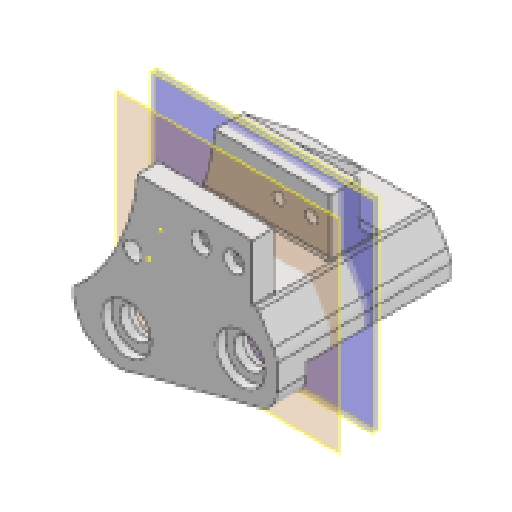
# Autodesk Inventor part: swingarmBaseV5
Saved by Autodesk Inventor 2025 (Build 290162000, 162)
## iProperties
Created: 2024-10-14
Part Number: swingarmBaseV5
Material: Generic
Document SubType Name: Modeling
Designer: derm
Density: 1 g/cm^3
Appearance: Default
Author: derm
Autodesk Inventor part; units mm, degrees
ref_plane "YZ Plane" through (0, 0, 0) normal (1, 0, 0) x (0, 1, 0)
ref_plane "XZ Plane" through (0, 0, 0) normal (0, 1, 0) x (-1, 0, 0)
ref_plane "XY Plane" through (0, 0, 0) normal (0, 0, 1) x (1, 0, 0)
sketch "Sketch1" plane through (0, 0, 0) normal (1, 0, 0) x (0, 1, 0)
  line L0 (-12.7635, 12.7635) -> (12.7635, 12.7635)
  line L1 (12.7635, 12.7635) -> (12.7635, -12.7635)
  line L2 (12.7635, -12.7635) -> (-12.7635, -12.7635)
  line L3 (-12.7635, -12.7635) -> (-12.7635, 12.7635)
  line L4 (-12.7635, 12.7635) -> (12.7635, -12.7635) construction
  line L5 (12.7635, 12.7635) -> (-12.7635, -12.7635) construction
  line L6 (19.1135, 19.1135) -> (-19.1135, 19.1135)
  line L7 (-19.1135, 19.1135) -> (-19.1135, -19.1135)
  line L8 (-19.1135, -19.1135) -> (19.1135, -19.1135)
  line L9 (19.1135, -19.1135) -> (19.1135, 19.1135)
  line L10 (12.7635, 19.1135) -> (12.7635, -19.1135)
  line L11 (-19.1135, -5.4793) -> (-46.5737, -5.4793)
  line L12 (-46.5737, -5.4793) -> (-46.5737, -19.1135)
  line L13 (-46.5737, -19.1135) -> (-19.1135, -19.1135)
  line L14 (-19.1135, -19.1135) -> (-19.1135, -5.4793)
  point P0 (0, 0)
  point P1 (12.7635, 12.7635)
  dimension "d1" = 25.527
  dimension "d2" = 6.35
  constraints: 30 end point, 6 parallel, 4 point on line, 3 perpendicular, 2 horizontal, 2 midpoint, 3 other
  measures "d1" distance of L1.end L2.end
  measures "d2" distance between parallel lines of L0 L6
extrude "Extrusion1" add sketch "Sketch1" along normal blind 50.8 contours L13 L12 L11 L7
sketch "Sketch2" plane through (0, -46.5737, -5.4793) normal (0, 0, 1) x (1, 0, 0)
  line L0 (0, 27.4602) -> (0, 0) projected
  line L1 (0, 0) -> (50.8, 0) projected
  line L2 (50.8, 27.4602) -> (50.8, 0) projected
  line L3 (0, 27.4602) -> (50.8, 27.4602) projected
  circle A0 centre (36.2123, 13.7301) radius 7
  point P0 (0, 46.5737)
  dimension "d5" = 14
  constraints: 1 centre point
  measures "d5" diameter of A0
extrude "Extrusion2" cut sketch "Sketch2" against normal through all contours A0
sketch "Sketch7" plane through (0, -46.5737, -5.4793) normal (0, 0, 1) x (1, 0, 0)
  circle A0 centre (36.2123, 13.7301) radius 7 projected
  circle A1 centre (36.2123, 13.7301) radius 11.1
  point P0 (0, 46.5737)
  dimension "d21" = 22.2
  constraints: 1 centre point, 1 coincident
  measures "d21" diameter of A1
extrude "Extrusion7" cut sketch "Sketch7" against normal blind 4
sketch "Sketch10" plane through (0, -46.5737, -19.1135) normal (0, 0, -1) x (-1, 0, 0)
  circle A0 centre (-36.2123, 13.7301) radius 7 projected
  line L0 (0, 0) -> (0, 27.4602) projected
  line L1 (0, 27.4602) -> (-50.8, 27.4602) projected
  line L2 (-50.8, 0) -> (-50.8, 27.4602) projected
  line L3 (0, 0) -> (-50.8, 0) projected
  circle A1 centre (-36.2123, 13.7301) radius 11
  point P0 (0, 46.5737)
  constraints: 1 centre point, 1 coincident
extrude "Extrusion10" cut sketch "Sketch10" against normal blind 5.5 contours A1
sketch "Sketch11" plane through (0, -46.5737, -5.4793) normal (0, 0, 1) x (1, 0, 0)
  circle A0 centre (36.2123, 13.7301) radius 11.1 projected
  circle A1 centre (8.2123, 21.7301) radius 2.6
  point P0 (0, 46.5737)
  dimension "d34" = 28
  dimension "d35" = 8
  dimension "d36" = 5.2
  constraints: 1 centre point
  measures "d34" horizontal distance of A0.centre A1.centre
  measures "d35" vertical distance of A0.centre A1.centre
  measures "d36" diameter of A1
extrude "Extrusion11" cut sketch "Sketch11" against normal through all contours A1
sketch "Sketch12" plane through (0, -19.1135, -5.4793) normal (0, 1, 0) x (1, 0, 0)
  line L0 (0, 13.6342) -> (0, 0) projected
  line L1 (0, 0) -> (50.8, 0) projected
  line L2 (50.8, 13.6342) -> (50.8, 0) projected
  line L3 (0, 13.6342) -> (50.8, 13.6342) projected
  point P0 (0, -5.4793)
extrude "Extrusion12" add sketch "Sketch12" along normal blind 10
sketch "Sketch13" plane through (50.8, -46.5737, -19.1135) normal (0, 0, -1) x (-1, 0, 0)
  circle A0 centre (42.5877, 21.7301) radius 2.6 projected
  circle A1 centre (14.5877, 13.7301) radius 11 projected
  line L0 (50.8, 0) -> (50.8, 37.4602) projected
  line L1 (0, 37.4602) -> (50.8, 37.4602) projected
  line L2 (0, 0) -> (0, 37.4602) projected
  line L3 (50.8, 0) -> (0, 0) projected
  line L4 (50.8, 0) -> (50.8, 37.4602) projected
  line L5 (0, 37.4602) -> (50.8, 37.4602)
  line L6 (50.8, 37.4602) -> (50.8, 28.3179)
  line L7 (50.8, 28.3179) -> (14.5877, 28.3179)
  line L8 (0, 28.3179) -> (0, 37.4602)
  arc A2 (14.5877, 28.3179) -> (0, 13.7301) centre (14.5877, 13.7301) ccw
  arc A3 (9.6596, 0) -> (19.5158, 0) centre (14.5877, 13.7301) ccw
  point P0 (50.8, 46.5737)
  constraints: 8 end point, 4 point on circle, 4 point on line, 2 centre point, 2 parallel, 2 tangent, 1 coincident, 1 horizontal, 1 perpendicular
extrude "Extrusion13" add sketch "Sketch13" along normal blind 26 contours L7 A2 L2 L1 L0
mirror "Mirror1" about plane through (25.4, -20.9786, -45.1135) normal (0, 0, -1)
fillet "Fillet5" [suppressed]
sketch "Sketch14" plane through (0, -9.1135, -5.4793) normal (0, 1, 0) x (1, 0, 0)
  line L0 (0, 0) -> (0, 79.2683) projected
  line L1 (0, 0) -> (50.8, 0) projected
  line L2 (50.8, 0) -> (50.8, 79.2683) projected
  line L3 (0, 79.2683) -> (50.8, 79.2683) projected
  circle A0 centre (-6.545, 39.6342) radius 15.197
  point P0 (0, -5.4793)
  constraints: 1 centre point
extrude "Extrusion14" cut sketch "Sketch14" against normal blind 26 contours A0 L0 | L0 A0
fillet "Fillet6" radius 10 2 edges at (0, -13.6847, -31.3981) (0, -13.6847, -58.8289)
sketch "Sketch15" plane through (50.8, -9.1135, -84.7477) normal (0, 0, -1) x (-1, 0, 0)
  line L0 (50.8, -37.4602) -> (0, -37.4602) projected
  line L1 (50.8, -37.4602) -> (50.8, 0) projected
  line L2 (50.8, 0) -> (0, 0) projected
  line L3 (0, -37.4602) -> (0, 0) projected
  circle A0 centre (42.5877, -15.7301) radius 2.6 projected
  circle A1 centre (14.5877, -23.7301) radius 11.1 projected
  circle A2 centre (-62.5324, 30.9366) radius 78.1359
  point P0 (50.8, 9.1135)
  point P1 (0, -15.9134)
  point P2 (9.2182, 0)
  constraints: 1 centre point
extrude "Extrusion15" cut sketch "Sketch15" against normal through all contours L3 L2 A2 picked at (1.1624, -8.9232)
thicken "Thicken1" operation add thickness 1.5 both sides no extend neighbours no toward (-0.9972038, -0.0747301, 0) faces at (50.7592, -31.7535, -36.4468)
fillet "Fillet7" radius 10 1 edges at (36.2123, -18.2559, -45.1135)
sketch "Sketch16" plane through (0, -9.1135, -5.4793) normal (0, 1, 0) x (1, 0, 0)
  line L0 (41.5818, 0) -> (41.5818, 79.2683) projected
  line L1 (0, 79.2683) -> (41.5818, 79.2683) projected
  line L2 (0, 58.6382) -> (0, 79.2683) projected
  arc A0 (0, 58.6382) -> (3.4337, 51.096) centre (10, 58.6382) ccw projected
  arc A1 (3.4337, 28.1723) -> (3.4337, 51.096) centre (-6.545, 39.6342) ccw projected
  arc A2 (3.4337, 28.1723) -> (0, 20.6301) centre (10, 20.6301) ccw projected
  line L3 (0, 0) -> (0, 20.6301) projected
  line L4 (0, 0) -> (41.5818, 0) projected
  line L5 (0, 0) -> (41.5818, 0)
  line L6 (41.5818, 0) -> (41.5818, 9.8)
  line L7 (41.5818, 9.8) -> (0, 9.8)
  line L8 (0, 9.8) -> (0, 0)
  line L9 (-402.451, 35.28) -> (156.349, 35.28) projected
  line L10 (8.0732, 35.48) -> (41.5818, 35.48)
  line L11 (5.8122, 48.48) -> (41.5818, 48.48)
  line L12 (41.5818, 48.48) -> (36.5818, 48.48)
  line L13 (36.5818, 48.48) -> (36.5818, 79.2683)
  line L14 (36.5818, 79.2683) -> (41.5818, 79.2683)
  line L15 (41.5818, 79.2683) -> (41.5818, 48.48)
  line L16 (5.8122, 48.48) -> (12.8122, 48.48)
  line L17 (12.8122, 48.48) -> (12.8122, 79.2683)
  line L18 (12.8122, 79.2683) -> (5.8122, 79.2683)
  line L19 (5.8122, 79.2683) -> (5.8122, 48.48)
  point P0 (0, -5.4793)
  point P1 (0, 9.8)
  dimension "d54" = 9.8
  dimension "d55" = 0.2
  dimension "d56" = 13
  dimension "d57" = 7
  dimension "d58" = 5
  constraints: 28 end point, 8 parallel, 5 point on line, 3 horizontal, 3 perpendicular, 2 point on circle
  measures "d54" distance between parallel lines of L4 L7
  measures "d55" distance between parallel lines of L9 L10
  measures "d56" distance between parallel lines of L10 L11
  measures "d57" distance between parallel lines of L19 L17
  measures "d58" distance between parallel lines of L0 L13
extrude "Extrusion16" add sketch "Sketch16" along normal blind 25.4 contours L4 L3 L7 L0 | L10 A1 L11 L0 | L19 L1 L17 L11
sketch "Sketch17" plane through (5.8122, -9.1135, -84.7477) normal (-1, 0, 0) x (0, 0, 1)
  line L0 (0, 0) -> (30.7883, 0) projected
  line L1 (0, 0) -> (0, 25.4) projected
  line L2 (30.7883, 25.4) -> (0, 25.4) projected
  line L3 (30.7883, 0) -> (30.7883, 25.4) projected
  line L4 (30.7883, 0) -> (0, 0) projected
  line L5 (30.7883, 0) -> (30.7883, 25.4) projected
  line L6 (0, 0) -> (30.7883, 25.4)
  point P0 (84.7477, 9.1135)
  constraints: 2 end point
extrude "Extrusion17" cut sketch "Sketch17" against normal blind 25.4 contours L1 L2 L6
fillet "Fillet8" radius 10 1 edges at (27.197, -9.1135, -53.9593)
sketch "Sketch18" plane through (-6.545, -18.2559, -45.1135) normal (0, -1, 0) x (1, 0, 0)
  line L0 (37.4895, 26) -> (37.4895, -26) projected
  line L1 (6.545, 26) -> (37.4895, 26) projected
  line L2 (6.545, 26) -> (6.545, 19.004) projected
  arc A0 (6.545, 19.004) -> (9.9788, 11.4619) centre (16.545, 19.004) ccw projected
  arc A1 (9.9788, -11.4619) -> (9.9788, 11.4619) centre (0, 0) ccw projected
  arc A2 (9.9788, -11.4619) -> (6.545, -19.004) centre (16.545, -19.004) ccw projected
  line L3 (6.545, -19.004) -> (6.545, -26) projected
  line L4 (6.545, -26) -> (37.4895, -26) projected
  line L5 (-395.906, 14.7702) -> (-395.906, 19.0981) projected
  line L6 (-395.906, 14.7702) -> (162.894, 14.7702) projected
  line L7 (162.894, 19.0981) -> (162.894, 14.7702) projected
  line L8 (-395.906, 19.0981) -> (162.894, 19.0981) projected
  circle A3 centre (29.9619, 16.9342) radius 2.6
  circle A4 centre (16.545, 16.9342) radius 2.6
  point P0 (6.545, 45.1135)
  dimension "d64" = 5.2
  constraints: 2 centre point
  measures "d64" diameter of A3
extrude "Extrusion18" cut sketch "Sketch18" against normal blind 25.4 contours A3 L6 L8 | L8 A3 | A3 L6 | A4 L8 | L8 A4 L6 | L6 A4
sketch "Sketch19" plane through (-6.545, -18.2559, -45.1135) normal (0, -1, 0) x (1, 0, 0)
  circle A0 centre (16.545, 16.9342) radius 2.6 projected
  circle A1 centre (29.9619, 16.9342) radius 2.6 projected
  circle A2 centre (16.545, 16.9342) radius 4
  circle A3 centre (29.9619, 16.9342) radius 4
  point P0 (6.545, 45.1135)
  dimension "d67" = 8
  dimension "d68" = 8
  constraints: 2 centre point, 2 coincident
  measures "d67" diameter of A3
  measures "d68" diameter of A2
extrude "Extrusion19" cut sketch "Sketch19" against normal blind 5
sketch "Sketch20" plane through (0, -46.5737, -84.7477) normal (0, 0, -1) x (-1, 0, 0)
  circle A0 centre (-8.2123, 21.7301) radius 2.6 projected
  circle A1 centre (-8.2123, 21.7301) radius 4.1
  point P0 (0, 46.5737)
  dimension "d71" = 8.2
  constraints: 1 centre point, 1 coincident
  measures "d71" diameter of A1
extrude "Extrusion20" cut sketch "Sketch20" against normal blind 8 contours A0 | A1
sketch "Sketch21" plane through (0, -46.5737, -5.4793) normal (0, 0, 1) x (1, 0, 0)
  circle A0 centre (8.2123, 21.7301) radius 2.6 projected
  circle A1 centre (8.2123, 21.7301) radius 4.1 projected
  circle A2 centre (8.2123, 21.7301) radius 3.5
  point P0 (0, 46.5737)
  dimension "d74" = 7
  constraints: 1 centre point, 1 coincident
  measures "d74" diameter of A2
extrude "Extrusion21" cut sketch "Sketch21" against normal blind 12 contours A2
sketch "Sketch22" plane through (41.5818, 16.2865, -53.9593) normal (0, 0, -1) x (-1, 0, 0)
  line L0 (444.0328, -10.536) -> (444.0328, -14.864) projected
  line L1 (444.0328, -10.536) -> (-114.7672, -10.536) projected
  line L2 (-114.7672, -14.864) -> (-114.7672, -10.536) projected
  line L3 (444.0328, -14.864) -> (-114.7672, -14.864) projected
  circle A0 centre (8.4648, -12.7) radius 2.6
  circle A1 centre (23.4097, -12.7) radius 2.6
  point P0 (41.5818, -16.2865)
  dimension "d77" = 5.2
  dimension "d78" = 5.2
  constraints: 2 centre point
  measures "d77" diameter of A0
  measures "d78" diameter of A1
extrude "Extrusion22" cut sketch "Sketch22" against normal through all contours A1 L3 L1 | L1 A1 | A1 L3 | A0 L3 L1 | L1 A0 | A0 L3
sketch "Sketch23" plane through (41.5818, 16.2865, -53.9593) normal (0, 0, -1) x (-1, 0, 0)
  circle A0 centre (23.4097, -12.7) radius 2.6 projected
  circle A1 centre (8.4648, -12.7) radius 2.6 projected
  line L0 (28.7696, -15.4) -> (0, -15.4) projected
  line L1 (28.7696, -15.4) -> (28.7696, 0) projected
  line L2 (0, 0) -> (28.7696, 0) projected
  line L3 (0, -15.4) -> (0, 0) projected
  circle A2 centre (8.4648, -12.7) radius 4.5
  circle A3 centre (23.4097, -12.7) radius 4.5
  point P0 (41.5818, -16.2865)
  dimension "d81" = 9
  dimension "d82" = 9
  constraints: 2 centre point, 2 coincident
  measures "d81" diameter of A3
  measures "d82" diameter of A2
extrude "Extrusion23" cut sketch "Sketch23" along normal mid plane 8 contours A0 | A3 L0 | L0 A3 | A2 L0 | L0 A2
ref_plane "Work Plane1" through (41.5818, -9.1135, -28.1193) normal (0, 0, -1) x (-1, 0, 0)
mirror "Mirror2" about plane through (41.5818, -9.1135, -28.1193) normal (0, 0, -1) of "Extrusion23"
fillet "Fillet9" [suppressed]
fillet "Fillet10" radius 5 1 edges at (50.8, -25.0269, -45.1135)
sketch "Sketch24" plane through (0, -46.5737, -84.7477) normal (0, -1, 0) x (1, 0, 0)
  line L0 (0, 79.2683) -> (0, 65.6342) projected
  line L1 (0, 65.6342) -> (50.8, 65.6342) projected
  line L2 (50.8, 79.2683) -> (50.8, 65.6342) projected
  line L3 (0, 79.2683) -> (50.8, 79.2683) projected
  line L4 (0, 0) -> (0, 13.6342) projected
  line L5 (0, 0) -> (50.8, 0) projected
  line L6 (50.8, 0) -> (50.8, 13.6342) projected
  line L7 (0, 13.6342) -> (50.8, 13.6342) projected
  point P0 (0, 84.7477)
extrude "Extrusion24" add sketch "Sketch24" along normal blind 5
sketch "Sketch25" plane through (41.5818, -9.1135, -84.7477) normal (0, 0, -1) x (-1, 0, 0)
  arc A0 (-8.2798, -14.634) -> (-9.2182, -17.5501) centre (-4.2182, -17.5501) ccw projected
  line L0 (-9.2182, -17.5501) -> (-9.2182, -42.4602) projected
  line L1 (41.5818, -42.4602) -> (-9.2182, -42.4602) projected
  line L2 (41.5818, -42.4602) -> (41.5818, 0) projected
  line L3 (41.5818, 0) -> (35.7696, 0) projected
  line L4 (35.7696, 0) -> (28.7696, 0) projected
  line L5 (28.7696, 0) -> (0, 0) projected
  arc A1 (-8.2798, -14.634) -> (0, 0) centre (-71.7506, 30.9366) ccw projected
  circle A2 centre (5.3695, -23.7301) radius 11.1 projected
  circle A3 centre (33.3695, -15.7301) radius 4.1 projected
  line L6 (5.3695, -42.4602) -> (41.5818, -27.5404)
  point P0 (41.5818, 9.1135)
  constraints: 2 end point, 2 point on line
extrude "Extrusion25" [suppressed]
fillet "Fillet12" [suppressed]
fillet "Fillet13" [suppressed]
chamfer "Chamfer2" distance 3 angle 45 5 edges at (0, -18.2559, -67.6155) (0.8988, -18.2559, -59.974) (8.652, -18.2559, -45.1135) (0.8988, -18.2559, -30.253) (0, -18.2559, -22.6115)
sketch "Sketch26" plane through (30.9444, -18.2559, -71.1135) normal (0, -1, 0) x (1, 0, 0)
  line L0 (-27.9444, 0) -> (-27.9444, 6.996) projected
  line L1 (-27.9444, 0) -> (0, 0) projected
  line L2 (0, 52) -> (0, 0) projected
  line L3 (-27.9444, 52) -> (0, 52) projected
  line L4 (-27.9444, 45.004) -> (-27.9444, 52) projected
  arc A0 (-27.9444, 45.004) -> (-25.5408, 39.7245) centre (-20.9444, 45.004) ccw projected
  arc A1 (-25.5408, 12.2755) -> (-25.5408, 39.7245) centre (-37.4895, 26) ccw projected
  arc A2 (-25.5408, 12.2755) -> (-27.9444, 6.996) centre (-20.9444, 6.996) ccw projected
  circle A3 centre (-7.5276, 42.9342) radius 4 projected
  circle A4 centre (-20.9444, 42.9342) radius 4 projected
  line L5 (-27.9444, 0) -> (-53.6411, 0)
  line L6 (-53.6411, 0) -> (-53.6411, 52)
  line L7 (-53.6411, 52) -> (-27.9444, 52)
  line L8 (-27.9444, 52) -> (-27.9444, 0)
  line L9 (10.6374, 55.8342) -> (-30.9444, 55.8342) projected
  line L10 (10.6374, 17.1542) -> (-18.1322, 17.1542) projected
  line L11 (-30.9444, 6.996) -> (-30.9444, -13.6342) projected
  line L12 (-30.9444, 55.8342) -> (-30.9444, 45.004) projected
  line L13 (-30.9444, 6.996) -> (-30.9444, 0) projected
  line L14 (-30.9444, 0) -> (-30.9444, 52)
  point P0 (-30.9444, 71.1135)
  point P1 (-30.9444, 54.8342)
  constraints: 10 end point, 2 parallel, 2 point on line, 1 horizontal, 1 perpendicular
extrude "Extrusion26" add sketch "Sketch26" against normal up to surface (9.1424 mm away) contours L5 L11 L14 L12 L7 L4 L8 L0 | L8 A0 A1 A2
sketch "Sketch27" plane through (0, -9.1135, -5.4793) normal (0, 1, 0) x (1, 0, 0)
  point P0 (0, -5.4793)
sketch "Sketch28" plane through (0, -9.1135, -5.4793) normal (0, 1, 0) x (1, 0, 0)
  line L0 (12.8122, 48.48) -> (5.8122, 48.48) projected
  arc A0 (8.0732, 35.48) -> (5.8122, 48.48) centre (-6.545, 39.6342) ccw projected
  line L1 (8.0732, 35.48) -> (41.5818, 35.48) projected
  line L2 (41.5818, 35.48) -> (41.5818, 48.48) projected
  line L3 (41.5818, 48.48) -> (12.8122, 48.48) projected
  line L4 (12.8122, 79.2683) -> (12.8122, 48.48) projected
  line L5 (5.8122, 79.2683) -> (12.8122, 79.2683) projected
  line L6 (5.8122, 48.48) -> (5.8122, 79.2683) projected
  line L7 (12.8122, 48.48) -> (5.8122, 48.48) projected
  line L8 (0, 9.8) -> (0, 79.2683) projected
  line L9 (0, 79.2683) -> (5.8122, 79.2683) projected
  line L10 (5.8122, 79.2683) -> (0, 79.2683)
  line L11 (8.0732, 35.48) -> (0, 35.48)
  point P0 (0, -5.4793)
  constraints: 4 end point, 1 horizontal, 1 perpendicular, 1 point on line
extrude "Extrusion27" add sketch "Sketch28" along normal up to surface (25.4 mm away) contours A0 L11 L8 L9 L6
sketch "Sketch29" plane through (5.8122, -9.1135, -84.7477) normal (1, 0, 0) x (0, 0, -1)
  line L0 (-30.7883, 25.4) -> (0, 0) projected
  line L1 (0, 0) -> (0, 25.4) projected
  line L2 (0, 25.4) -> (-30.7883, 25.4) projected
  point P0 (-84.7477, 9.1135)
extrude "Extrusion28" cut sketch "Sketch29" against normal blind 10
sketch "Sketch30" plane through (0, 0, 0) normal (-1, 0, 0) x (0, 0, 1)
  line L0 (-53.9593, 16.2865) -> (-84.7477, -9.1135) projected
  line L1 (-84.7477, -51.5737) -> (-84.7477, -9.1135) projected
  line L2 (-71.1135, -51.5737) -> (-84.7477, -51.5737) projected
  line L3 (-71.1135, -51.5737) -> (-71.1135, -18.2559) projected
  line L4 (-19.1135, -18.2559) -> (-71.1135, -18.2559) projected
  line L5 (-19.1135, -18.2559) -> (-19.1135, -51.5737) projected
  line L6 (-5.4793, -51.5737) -> (-19.1135, -51.5737) projected
  line L7 (-5.4793, -51.5737) -> (-5.4793, 16.2865) projected
  line L8 (-15.2793, 16.2865) -> (-5.4793, 16.2865) projected
  line L9 (-15.2793, -9.1135) -> (-15.2793, 16.2865) projected
  line L10 (-15.2793, -9.1135) -> (-40.9593, -9.1135) projected
  line L11 (-40.9593, -9.1135) -> (-40.9593, 16.2865) projected
  line L12 (-40.9593, 16.2865) -> (-53.9593, 16.2865) projected
  line L13 (-40.9593, -9.1135) -> (-63.9593, -9.1135) projected
  line L14 (-84.7477, -9.1135) -> (-63.9593, -9.1135) projected
  line L15 (-40.9593, -9.1135) -> (-84.7477, -9.1135)
  line L16 (-84.7477, -9.1135) -> (-5.4793, -9.1135)
  point P0 (0, 0)
  constraints: 4 end point, 2 point on line, 1 collinear
extrude "Extrusion29" add sketch "Sketch30" along normal blind 20 contours L14 L13 L10 L16 L7 L6 L5 L4 L3 L2 L1
pattern_linear "Rectangular Pattern1" [suppressed]
sketch "Sketch31" plane through (0.7123, -24.8436, -17.4793) normal (0, 0, 1) x (1, 0, 0)
  circle A0 centre (0, 0) radius 2.6 projected
  point P0 (-0.7123, 24.8436)
extrude "Extrusion30" [suppressed]
sketch "Sketch32" plane through (0, -9.1135, -5.4793) normal (0, 1, 0) x (1, 0, 0)
  line L0 (-20, 65.6342) -> (30.9444, 65.6342) projected
  line L1 (30.9444, 13.6342) -> (30.9444, 65.6342) projected
  line L2 (-20, 13.6342) -> (30.9444, 13.6342) projected
  line L3 (-20, 65.6342) -> (-20, 13.6342) projected
  circle A0 centre (23.4168, 22.7) radius 4 projected
  circle A1 centre (10, 22.7) radius 4 projected
  line L4 (-20, 65.6342) -> (-20, 13.6342) projected
  arc A2 (-20, 13.6342) -> (-20, 65.6342) centre (-29.611, 39.6342) ccw
  point P0 (0, -5.4793)
  constraints: 2 point on circle, 1 centre point
extrude "Extrusion31" cut sketch "Sketch32" against normal blind 10 contours A2 L3
sketch "Sketch33" plane through (0, -9.1135, -5.4793) normal (0, 1, 0) x (1, 0, 0)
  line L0 (0, 9.8) -> (0, 0) projected
  line L1 (0, 0) -> (41.5818, 0) projected
  line L2 (41.5818, 0) -> (41.5818, 9.8) projected
  line L3 (41.5818, 9.8) -> (0, 9.8) projected
  line L4 (12.8122, 48.48) -> (0, 48.48) projected
  line L5 (0, 9.8) -> (0, 0) projected
  line L6 (41.5818, 35.48) -> (0, 35.48) projected
  line L7 (41.5818, 35.48) -> (41.5818, 48.48) projected
  line L8 (41.5818, 48.48) -> (12.8122, 48.48) projected
  arc A0 (-20, 13.6342) -> (-20, 65.6342) centre (-29.611, 39.6342) ccw projected
  line L9 (-20, 0) -> (-20, 13.6342) projected
  line L10 (0, 0) -> (-20, 0) projected
  line L11 (0, 9.8) -> (0, 0) projected
  line L12 (0, 9.8) -> (41.5818, 9.8) projected
  line L13 (41.5818, 9.8) -> (41.5818, 35.48) projected
  line L14 (41.5818, 35.48) -> (0, 35.48) projected
  line L15 (0, 79.2683) -> (0, 35.48) projected
  line L16 (0, 79.2683) -> (-20, 79.2683) projected
  line L17 (-20, 65.6342) -> (-20, 79.2683) projected
  circle A1 centre (10, 22.7) radius 2.6 projected
  circle A2 centre (23.4168, 22.7) radius 2.6 projected
  line L18 (0, 9.8) -> (-20, 9.8)
  line L19 (0, 48.48) -> (-3.3408, 48.48)
  line L20 (0, 35.48) -> (-2.2046, 35.48)
  line L21 (0, 0) -> (41.5818, 0) projected
  line L22 (41.5818, 0) -> (41.5818, 9.8) projected
  line L23 (41.5818, 9.8) -> (0, 9.8) projected
  line L24 (0, 35.48) -> (0, 48.48) projected
  point P0 (0, -5.4793)
  constraints: 6 end point, 2 point on circle, 2 point on line, 1 parallel, 1 perpendicular
extrude "Extrusion32" add sketch "Sketch33" along normal up to surface (25.4 mm away) contours L3 L2 L1 L0 | L0 L10 L9 L18
fillet "Fillet14" radius 1 2 edges at (10.7909, -9.1135, -15.2793) (20.7909, -9.1135, -40.9593)
sketch "Sketch34" plane through (41.5818, -9.1135, -84.7477) normal (0, 0, -1) x (-1, 0, 0)
  line L0 (41.5818, 0) -> (28.7696, 0) projected
  line L1 (28.7696, 0) -> (0, 0) projected
  arc A0 (-8.2798, -14.634) -> (0, 0) centre (-71.7506, 30.9366) ccw projected
  arc A1 (-8.2798, -14.634) -> (-9.2182, -17.5501) centre (-4.2182, -17.5501) ccw projected
  line L2 (-9.2182, -17.5501) -> (-9.2182, -42.4602) projected
  line L3 (-9.2182, -42.4602) -> (61.5818, -42.4602) projected
  line L4 (61.5818, 0) -> (61.5818, -42.4602) projected
  line L5 (41.5818, 0) -> (61.5818, 0) projected
  circle A2 centre (33.3695, -15.7301) radius 4.1 projected
  line L6 (0, 10) -> (0, 0) projected
  line L7 (0, 0) -> (-2.106, 0)
  line L8 (-2.106, 0) -> (-11.1734, -14.634)
  line L9 (-11.1734, -14.634) -> (-11.1734, -42.4602)
  line L10 (-11.1734, -42.4602) -> (-9.2182, -42.4602)
  point P0 (41.5818, 9.1135)
  constraints: 8 end point, 2 perpendicular, 1 horizontal
extrude "Extrusion33" add sketch "Sketch34" against normal up to surface (79.2683 mm away) contours A0 A1 L2 L10 L9 L8 L7
sketch "Sketch35" plane through (50.8, -51.5737, -71.1135) normal (-1, 0, 0) x (0, 0, 1)
  line L0 (0, 0) -> (0, 18.7301) projected
  line L1 (0, 0) -> (52, 0) projected
  line L2 (52, 18.7301) -> (52, 0) projected
  line L3 (52, 18.7301) -> (0, 18.7301) projected
  point P0 (71.1135, 51.5737)
extrude "Extrusion34" cut sketch "Sketch35" against normal blind 10
fillet "Fillet15" [suppressed]
sketch "Sketch39" plane through (41.5818, -9.1135, -5.4793) normal (0, 0, 1) x (1, 0, 0)
  point P0 (-41.5818, 9.1135)
sketch "Sketch41" plane through (0, -46.5737, -76.7477) normal (0, 0, -1) x (-1, 0, 0)
  circle A0 centre (6.7877, 21.7301) radius 2.6 projected
  point P0 (0, 46.5737)
extrude "Extrusion39" cut sketch "Sketch41" against normal blind 10
sketch "Sketch42" plane through (-20, 0, 0) normal (-1, 0, 0) x (0, 0, 1)
  line L0 (-71.1135, -18.2559) -> (-71.1135, -9.1135) projected
  line L1 (-71.1135, -9.1135) -> (-84.7477, -9.1135) projected
  line L2 (-84.7477, -9.1135) -> (-84.7477, -51.5737) projected
  line L3 (-84.7477, -51.5737) -> (-71.1135, -51.5737) projected
  line L4 (-71.1135, -51.5737) -> (-71.1135, -18.2559) projected
  line L5 (-13.6135, -43.8436) -> (-13.6135, -21.8436) projected
  line L6 (-19.1135, -9.1135) -> (-19.1135, -18.2559) projected
  line L7 (-19.1135, -18.2559) -> (-19.1135, -51.5737) projected
  line L8 (-19.1135, -51.5737) -> (-5.4793, -51.5737) projected
  line L9 (-5.4793, -51.5737) -> (-5.4793, 16.2865) projected
  line L10 (-5.4793, 16.2865) -> (-15.2793, 16.2865) projected
  line L11 (-15.2793, -8.1135) -> (-15.2793, 16.2865) projected
  arc A0 (-16.2793, -9.1135) -> (-15.2793, -8.1135) centre (-16.2793, -8.1135) ccw projected
  line L12 (-16.2793, -9.1135) -> (-19.1135, -9.1135) projected
  line L13 (-84.7477, -23.7475) -> (-84.7477, -51.5737) projected
  line L14 (-84.7477, -51.5737) -> (-71.1135, -51.5737)
  line L15 (-71.1135, -51.5737) -> (-71.1135, -67.9032)
  line L16 (-71.1135, -67.9032) -> (-84.7477, -67.9032)
  line L17 (-84.7477, -67.9032) -> (-84.7477, -51.5737)
  line L18 (-19.1135, -51.5737) -> (-5.4793, -51.5737)
  line L19 (-5.4793, -51.5737) -> (-5.4793, -67.9032)
  line L20 (-5.4793, -67.9032) -> (-19.1135, -67.9032)
  line L21 (-19.1135, -67.9032) -> (-19.1135, -51.5737)
  point P0 (0, 0)
  constraints: 16 end point, 4 parallel, 2 horizontal, 2 perpendicular, 1 point on line
extrude "Extrusion40" add sketch "Sketch42" against normal up to surface (72.7552 mm away) contours L15 L16 L17 L3 | L8 L19 L20 L21
sketch "Sketch46" plane through (-20, 0, 0) normal (-1, 0, 0) x (0, 0, 1)
  line L0 (-71.1135, -18.2559) -> (-71.1135, -9.1135) projected
  line L1 (-71.1135, -9.1135) -> (-84.7477, -9.1135) projected
  line L2 (-84.7477, -9.1135) -> (-84.7477, -67.9032) projected
  line L3 (-84.7477, -67.9032) -> (-71.1135, -67.9032) projected
  line L4 (-71.1135, -67.9032) -> (-71.1135, -18.2559) projected
  line L5 (-19.1135, -9.1135) -> (-19.1135, -18.2559) projected
  line L6 (-19.1135, -18.2559) -> (-19.1135, -67.9032) projected
  line L7 (-19.1135, -67.9032) -> (-5.4793, -67.9032) projected
  line L8 (-5.4793, -67.9032) -> (-5.4793, 16.2865) projected
  line L9 (-5.4793, 16.2865) -> (-15.2793, 16.2865) projected
  line L10 (-15.2793, -8.1135) -> (-15.2793, 16.2865) projected
  arc A0 (-16.2793, -9.1135) -> (-15.2793, -8.1135) centre (-16.2793, -8.1135) ccw projected
  line L11 (-16.2793, -9.1135) -> (-19.1135, -9.1135) projected
  point P0 (0, 0)
extrude "Extrusion44" add sketch "Sketch46" along normal blind 20
sketch "Sketch43" plane through (12.8122, -9.1135, -84.7477) normal (0, 0, -1) x (-1, 0, 0)
  line L0 (12.8122, 0) -> (0, 0) projected
  line L1 (0, 0) -> (-30.8757, 0) projected
  line L2 (-30.8757, 0) -> (-39.943, -14.634) projected
  line L3 (-39.943, -14.634) -> (-39.943, -58.7897) projected
  line L4 (52.8122, -58.7897) -> (-39.943, -58.7897) projected
  line L5 (12.8122, 0) -> (52.8122, 0) projected
  circle A0 centre (4.5999, -15.7301) radius 4.1 projected
  circle A1 centre (28.5229, -37.9631) radius 11.1
  line L6 (52.8122, 0) -> (52.8122, -58.7897) projected
  point P0 (12.8122, 9.1135)
  dimension "d143" = 22.2
  constraints: 1 centre point
  measures "d143" diameter of A1
extrude "Extrusion41" cut sketch "Sketch43" against normal up to surface (4 mm away) contours A1
sketch "Sketch44" plane through (-15.7107, -47.0766, -80.7477) normal (0, 0, -1) x (-1, 0, 0)
  circle A0 centre (0, 0) radius 11.1 projected
  circle A1 centre (0, 0) radius 7
  point P0 (-15.7107, 47.0766)
  dimension "d148" = 14
  constraints: 1 centre point, 1 coincident
  measures "d148" diameter of A1
extrude "Extrusion42" cut sketch "Sketch44" against normal up to surface (9.6342 mm away) contours A1
sketch "Sketch45" plane through (-20, -18.2559, -71.1135) normal (0, 0, 1) x (1, 0, 0)
  circle A0 centre (4.2893, -28.8208) radius 7 projected
  circle A1 centre (4.2893, -28.8208) radius 11.1 projected
  point P0 (20, 18.2559)
extrude "Extrusion43" cut sketch "Sketch45" against normal up to surface (5.5 mm away)
ref_plane "Work Plane2" through (12.8122, -9.1135, -45.1135) normal (0, 0, -1) x (-1, 0, 0)
mirror "Mirror3" about plane through (12.8122, -9.1135, -45.1135) normal (0, 0, -1) of "Extrusion43", "Extrusion42", "Extrusion41", "Extrusion20", "Extrusion21", "Extrusion11"
sketch "Sketch47" plane through (41.5818, -9.1135, -5.4793) normal (0, 0, 1) x (1, 0, 0)
  line L0 (11.1734, -58.7897) -> (-81.5818, -58.7897) projected
  line L1 (11.1734, -14.634) -> (11.1734, -58.7897) projected
  line L2 (2.106, 0) -> (11.1734, -14.634) projected
  line L3 (0, 0) -> (2.106, 0) projected
  line L4 (0, 0) -> (0, 25.4) projected
  line L5 (0, 25.4) -> (-81.5818, 25.4) projected
  line L6 (-81.5818, -58.7897) -> (-81.5818, 25.4) projected
  circle A0 centre (-5.3695, -23.7301) radius 11.1 projected
  circle A1 centre (-57.2925, -37.9631) radius 11.1 projected
  circle A2 centre (-33.3695, -15.7301) radius 4.1 projected
  line L7 (-81.5818, -58.7897) -> (11.1734, -58.7897)
  line L8 (11.1734, -14.634) -> (11.1734, -58.7897)
  line L9 (-81.5818, -58.7897) -> (11.1734, -58.7897) projected
  line L10 (-73.3351, -58.7897) -> (11.1734, -36.7118)
  point P0 (-41.5818, 9.1135)
  point P1 (11.1734, -36.7118)
  point P2 (-73.3351, -58.7897)
  constraints: 6 end point, 2 collinear, 1 midpoint, 1 point on line
extrude "Extrusion45" cut sketch "Sketch47" against normal through all contours L0 L10 L1
sketch "Sketch49" plane through (12.8122, -9.1135, -84.7477) normal (0, 0, -1) x (-1, 0, 0)
  circle A0 centre (4.5999, -15.7301) radius 4.1 projected
  circle A1 centre (-23.4001, -23.7301) radius 11.1 projected
  line L0 (-39.943, -36.7118) -> (44.5655, -58.7897) projected
  line L1 (52.8122, -58.7897) -> (44.5655, -58.7897) projected
  line L2 (52.8122, 0) -> (52.8122, -58.7897) projected
  line L3 (12.8122, 0) -> (52.8122, 0) projected
  line L4 (12.8122, 0) -> (0, 0) projected
  line L5 (0, 0) -> (-30.8757, 0) projected
  line L6 (-30.8757, 0) -> (-39.943, -14.634) projected
  line L7 (-39.943, -14.634) -> (-39.943, -36.7118) projected
  circle A2 centre (28.5229, -37.9631) radius 11.1 projected
  circle A3 centre (25.5999, -5.7301) radius 2.6
  circle A4 centre (4.5999, -15.7301) radius 3.5 projected
  circle A5 centre (4.5999, -15.7301) radius 2.6 projected
  point P0 (12.8122, 9.1135)
  dimension "d162" = 21
  dimension "d164" = 10
  constraints: 1 centre point, 1 equal radius
  measures "d162" horizontal distance of A3.centre A0.centre
  measures "d164" vertical distance of A3.centre A0.centre
extrude "Extrusion46" cut sketch "Sketch49" against normal through all contours A3
sketch "Sketch50" plane through (12.8122, -9.1135, -84.7477) normal (0, 0, -1) x (-1, 0, 0)
  circle A0 centre (4.5999, -15.7301) radius 4.1 projected
  circle A1 centre (25.5999, -5.7301) radius 2.6 projected
  circle A2 centre (25.5999, -5.7301) radius 4.1
  point P0 (12.8122, 9.1135)
  dimension "d165" = 8.2
  constraints: 1 centre point, 1 coincident
  measures "d165" diameter of A2
extrude "Extrusion47" cut sketch "Sketch50" against normal blind 7 contours A2
ref_plane "Work Plane3" through (12.8122, -9.1135, -45.1135) normal (0, 0, -1) x (-1, 0, 0)
mirror "Mirror4" about plane through (12.8122, -9.1135, -45.1135) normal (0, 0, -1) of "Extrusion47"
ref_plane "Work Plane4" through (41.5818, -9.1135, -29.7193) normal (0, 0, 1) x (1, 0, 0)
mirror "Mirror5" about plane through (41.5818, -9.1135, -29.7193) normal (0, 0, 1) of "Extrusion23", "Extrusion22"
sketch "Sketch51" plane through (30.9444, -18.2559, -71.1135) normal (0, -1, 0) x (1, 0, 0)
  circle A0 centre (-20.9444, 42.9342) radius 4 projected
  circle A1 centre (-7.5276, 42.9342) radius 4 projected
  arc A2 (-50.9444, 0) -> (-50.9444, 52) centre (-60.5555, 26) ccw projected
  line L0 (-50.9444, 0) -> (0, 0) projected
  line L1 (0, 52) -> (0, 0) projected
  line L2 (-50.9444, 52) -> (0, 52) projected
  line L3 (-20.5332, 35.9231) -> (-45.3247, 35.9231)
  line L4 (-45.3247, 35.9231) -> (-45.3247, 11.5388)
  line L5 (-45.3247, 11.5388) -> (-20.5332, 11.5388)
  line L6 (-20.5332, 11.5388) -> (-20.5332, 35.9231)
  line L7 (-20.5332, 35.9231) -> (-45.3247, 11.5388) construction
  line L8 (-45.3247, 35.9231) -> (-20.5332, 11.5388) construction
  line L9 (-32.929, 11.5388) -> (-32.929, 35.9231)
  point P0 (-30.9444, 71.1135)
  point P1 (-32.929, 23.7309)
  point P2 (-34.6729, 35.9231)
  point P3 (-36.9071, 11.5388)
  constraints: 14 end point, 4 midpoint, 2 parallel, 1 horizontal, 1 perpendicular, 1 point on circle, 1 other
sketch "Sketch52" plane through (30.9444, -18.2559, -19.1135) normal (0, 0, -1) x (-1, 0, 0)
  circle A0 centre (22.7322, -6.5877) radius 2.6 projected
  circle A1 centre (-5.2678, -14.5877) radius 11 projected
  line L0 (-21.8108, -27.5694) -> (62.6977, -49.6473) projected
  line L1 (62.6977, -49.6473) -> (70.9444, -49.6473) projected
  line L2 (70.9444, 9.1424) -> (70.9444, -49.6473) projected
  line L3 (50.9444, 9.1424) -> (70.9444, 9.1424) projected
  line L4 (50.9444, 9.1424) -> (50.9444, 0) projected
  line L5 (50.9444, 0) -> (0, 0) projected
  arc A2 (0, 0) -> (-5.2678, -1.5) centre (0, -10) ccw projected
  arc A3 (-5.2678, -1.5) -> (-18.3556, -14.5877) centre (-5.2678, -14.5877) ccw projected
  line L6 (-18.3556, -14.5877) -> (-21.8108, -14.5877) projected
  line L7 (-21.8108, -27.5694) -> (-21.8108, -14.5877) projected
  circle A4 centre (46.6552, -28.8208) radius 11.1 projected
  spline S0 degree 2 poles (46.3322, 3.4123) (46.3322, 7.9156) (42.4322, 5.6639) (38.5322, 3.4123) (42.4322, 1.1606) (46.3322, -1.0911) (46.3322, 3.4123) knots 0 0 0 0.333333 0.333333 0.666667 0.666667 1 1 1 weights 1 0.5 1 0.5 1 0.5 1 projected
  line L8 (50.9444, 0) -> (50.9444, 0) projected
  line L9 (50.9444, 9.1424) -> (50.9444, 0) projected
  line L10 (50.9444, 9.1424) -> (50.9444, 9.1424) projected
  line L11 (50.9444, 0) -> (50.9444, 9.1424) projected
  line L12 (36.9815, 0) -> (36.9815, 9.1424)
  line L13 (36.9815, 9.1424) -> (50.9444, 9.1424)
  line L14 (-10.6374, 9.1424) -> (70.9444, 9.1424) projected
  line L15 (34.7197, 4) -> (34.7197, 9.1424)
  line L16 (50.9444, 9.1424) -> (60.5203, 9.1424)
  line L17 (60.5203, 9.1424) -> (60.5203, 0)
  line L18 (60.5203, 0) -> (50.9444, 0)
  line L19 (50.9444, 0) -> (50.9444, 9.1424)
  line L20 (27.5865, 9.1424) -> (27.5865, 0)
  point P0 (30.9444, 18.2559)
  point P1 (60.5203, 9.1424)
  constraints: 16 end point, 3 point on line, 2 parallel, 2 perpendicular, 1 collinear, 1 horizontal, 1 vertical, 3 other
extrude "Extrusion49" add sketch "Sketch52" along normal blind 21 contours L17 L18 L4 L3 | L4 L5 L12 L13 | L20 L14 L12 L5
ref_plane "Work Plane5" through (14.8297, -14.2559, -47.3826) normal (0, 0, -1) x (-1, 0, 0)
mirror "Mirror6" about plane through (14.8297, -14.2559, -47.3826) normal (0, 0, -1) of "Extrusion49"
sketch "Sketch53" plane through (30.9444, -18.2559, -71.1135) normal (0, -1, 0) x (1, 0, 0)
  line L0 (-60.5203, 0) -> (0, 0) projected
  line L1 (0, 52) -> (0, 0) projected
  line L2 (-60.5203, 52) -> (0, 52) projected
  line L3 (-60.5203, 52) -> (-60.5203, 31) projected
  line L4 (-33.2906, 31) -> (-60.5203, 31) projected
  line L5 (-34.5286, 16.4619) -> (-60.5203, 16.4619) projected
  line L6 (-60.5203, 0) -> (-60.5203, 16.4619) projected
  circle A0 centre (-7.5276, 42.9342) radius 4 projected
  circle A1 centre (-20.9444, 42.9342) radius 4 projected
  line L7 (0, 52) -> (5.2678, 52) projected
  line L8 (0, 52) -> (0, 0) projected
  line L9 (5.2678, 0) -> (0, 0) projected
  line L10 (5.2678, 52) -> (5.2678, 0) projected
  line L11 (5.2678, 52) -> (18.3556, 52) projected
  line L12 (5.2678, 52) -> (5.2678, 0) projected
  line L13 (18.3556, 0) -> (5.2678, 0) projected
  line L14 (18.3556, 52) -> (18.3556, 0) projected
  arc A2 (-34.5286, 16.4619) -> (-33.2906, 31) centre (-60.5555, 26) ccw projected
  point P0 (-30.9444, 71.1135)
extrude "Extrusion50" [suppressed]
sketch "Sketch54" plane through (12.8122, -9.1135, -84.7477) normal (0, 0, -1) x (-1, 0, 0)
  circle A0 centre (25.5999, -5.7301) radius 4.1 projected
  circle A1 centre (4.5999, -15.7301) radius 4.1 projected
  circle A2 centre (-23.4001, -23.7301) radius 11.1 projected
  line L0 (-39.943, -36.7118) -> (44.5655, -58.7897) projected
  line L1 (52.8122, -58.7897) -> (44.5655, -58.7897) projected
  line L2 (52.8122, 0) -> (52.8122, -58.7897) projected
  line L3 (12.8122, 0) -> (52.8122, 0) projected
  line L4 (12.8122, 0) -> (0, 0) projected
  line L5 (0, 0) -> (-30.8757, 0) projected
  line L6 (-30.8757, 0) -> (-39.943, -14.634) projected
  line L7 (-39.943, -14.634) -> (-39.943, -36.7118) projected
  circle A3 centre (28.5229, -37.9631) radius 11.1 projected
  line L8 (52.8122, -16.7272) -> (-19.9536, -41.9341)
  point P0 (12.8122, 9.1135)
  constraints: 2 end point, 2 point on line
extrude "Extrusion51" cut sketch "Sketch54" against normal blind 15 contours L8 L2 L1 L0 | A3
fillet "Fillet21" radius 2 1 edges at (43.6878, -9.1135, -45.1135)
fillet "Fillet22" radius 10 1 edges at (52.7552, -23.7475, -45.1135)
fillet "Fillet23" radius 10 2 edges at (52.7552, -45.8253, -12.2964) (52.7552, -45.8253, -77.9306)
fillet "Fillet24" radius 40 1 edges at (32.7657, -51.0476, -77.9306)
fillet "Fillet26" radius 20 2 edges at (-31.7533, -67.9032, -12.2964) (-40, -67.9032, -12.2964)
sketch "Sketch55" plane through (52.7552, -32.8436, -19.1135) normal (0, 0, -1) x (-1, 0, 0)
  circle A0 centre (16.5429, 0) radius 11.1 projected
  circle A1 centre (44.5429, 8) radius 4.1 projected
  circle A2 centre (65.5429, 18) radius 4.1 projected
  arc A3 (8.2503, -15.1371) -> (31.4541, -14.2324) centre (18.361, 23.564) ccw projected
  line L0 (31.4541, -14.2324) -> (92.7552, 7.003) projected
  line L1 (92.7552, 23.7301) -> (92.7552, 7.003) projected
  line L2 (52.7552, 23.7301) -> (92.7552, 23.7301) projected
  line L3 (52.7552, 23.7301) -> (39.943, 23.7301) projected
  line L4 (39.943, 23.7301) -> (10.1809, 23.7301) projected
  arc A4 (10.1809, 23.7301) -> (8.4808, 22.7835) centre (10.1809, 21.7301) ccw projected
  line L5 (8.4808, 22.7835) -> (1.4995, 11.5162) projected
  arc A5 (1.4995, 11.5162) -> (0, 6.2492) centre (10, 6.2492) ccw projected
  line L6 (0, 6.2492) -> (0, -5.2586) projected
  arc A6 (0, -5.2586) -> (7.4723, -14.9338) centre (10, -5.2586) ccw projected
  line L7 (7.4723, -14.9338) -> (8.2503, -15.1371) projected
  line L8 (82.331, 23.7301) -> (82.331, 14.5877) projected
  line L9 (82.331, 23.7301) -> (92.7552, 23.7301)
  line L10 (92.7552, 23.7301) -> (92.7552, 7.003)
  line L11 (92.7552, 7.003) -> (82.331, 7.003)
  line L12 (82.331, 7.003) -> (82.331, 23.7301)
  point P0 (52.7552, 32.8436)
  point P1 (82.331, 12.5877)
  constraints: 8 end point, 2 parallel, 1 horizontal, 1 perpendicular
extrude "Extrusion52" add sketch "Sketch55" along normal up to surface (52 mm away) contours L11 L12 L8 L2 L1
sketch "Sketch56" plane through (12.8122, -9.1135, -84.7477) normal (0, 0, -1) x (-1, 0, 0)
  circle A0 centre (-23.4001, -23.7301) radius 11.1 projected
  circle A1 centre (4.5999, -15.7301) radius 4.1 projected
  circle A2 centre (25.5999, -5.7301) radius 4.1 projected
  arc A3 (-31.6927, -38.8672) -> (-8.4889, -37.9626) centre (-21.582, -0.1661) ccw projected
  line L0 (-8.4889, -37.9626) -> (52.8122, -16.7272) projected
  line L1 (52.8122, 0) -> (52.8122, -16.7272) projected
  line L2 (12.8122, 0) -> (52.8122, 0) projected
  line L3 (12.8122, 0) -> (0, 0) projected
  line L4 (0, 0) -> (-29.7621, 0) projected
  arc A4 (-29.7621, 0) -> (-31.4622, -0.9466) centre (-29.7621, -2) ccw projected
  line L5 (-31.4622, -0.9466) -> (-38.4435, -12.2139) projected
  arc A5 (-38.4435, -12.2139) -> (-39.943, -17.4809) centre (-29.943, -17.4809) ccw projected
  line L6 (-39.943, -17.4809) -> (-39.943, -28.9887) projected
  arc A6 (-39.943, -28.9887) -> (-32.4707, -38.664) centre (-29.943, -28.9887) ccw projected
  line L7 (-32.4707, -38.664) -> (-31.6927, -38.8672) projected
  line L8 (-39.943, -23.7301) -> (32.5965, -23.7301)
  point P0 (12.8122, 9.1135)
  constraints: 2 end point, 1 horizontal, 1 point on line
extrude "Extrusion53" cut sketch "Sketch56" against normal up to surface (13.6342 mm away) contours L8 L0 A3 L7 A6 L6 A0 | A0 L8 picked at (-24.7121, -27.1897)
sketch "Sketch57" plane through (12.8122, -9.1135, -84.7477) normal (0, 0, -1) x (-1, 0, 0)
  arc A0 (-12.3001, -23.7301) -> (-34.5001, -23.7301) centre (-23.4001, -23.7301) ccw projected
  circle A1 centre (-23.4001, -23.7301) radius 11.8982
  line L0 (-35.2982, -23.7301) -> (-11.5019, -23.7301)
  line L1 (32.5965, -23.7301) -> (-12.4001, -23.7301) projected
  point P0 (12.8122, 9.1135)
  point P1 (-28.7696, 25.4)
  constraints: 2 end point, 2 point on circle, 1 centre point, 1 coincident, 1 point on line
extrude "Extrusion54" add sketch "Sketch57" against normal up to surface (8.1342 mm away) contours L0 A0 | A0 L0 A1
sketch "Sketch58" plane through (12.8122, -9.1135, -84.7477) normal (0, 0, -1) x (-1, 0, 0)
  circle A0 centre (4.5999, -15.7301) radius 4.1 projected
  circle A1 centre (25.5999, -5.7301) radius 4.1 projected
  line L0 (-39.943, -23.7301) -> (32.5965, -23.7301) projected
  line L1 (32.5965, -23.7301) -> (52.8122, -16.7272) projected
  line L2 (52.8122, 0) -> (52.8122, -16.7272) projected
  line L3 (12.8122, 0) -> (52.8122, 0) projected
  line L4 (12.8122, 0) -> (0, 0) projected
  line L5 (0, 0) -> (-29.7621, 0) projected
  arc A2 (-29.7621, 0) -> (-31.4622, -0.9466) centre (-29.7621, -2) ccw projected
  line L6 (-31.4622, -0.9466) -> (-38.4435, -12.2139) projected
  arc A3 (-38.4435, -12.2139) -> (-39.943, -17.4809) centre (-29.943, -17.4809) ccw projected
  line L7 (-39.943, -17.4809) -> (-39.943, -23.7301) projected
  circle A4 centre (110.762, 31.5977) radius 87.2843
  point P0 (12.8122, 9.1135)
  dimension "d189" = 57.9498
  dimension "d190" = 31.5977
  constraints: 1 centre point
  measures "d189" distance from line of A4.centre L2
  measures "d190" distance from line of A4.centre L3
extrude "Extrusion55" cut sketch "Sketch58" against normal through all contours A4 L3 L2 L1 | L1 L2 L3 A4
extrude "Extrusion57" cut sketch "Sketch51" against normal blind 4 contours A2 L9 L5 | A2 L9 L3 L6 L5 | A2 L3 L9
sketch "Sketch59" plane through (12.8122, -9.1135, -84.7477) normal (0, 0, -1) x (-1, 0, 0)
  arc A0 (29.3978, 0) -> (40.9756, -20.8275) centre (110.762, 31.5977) ccw projected
  line L0 (12.8122, 0) -> (29.3978, 0) projected
  line L1 (12.8122, 0) -> (0, 0) projected
  line L2 (0, 0) -> (-29.7621, 0) projected
  arc A1 (-29.7621, 0) -> (-31.4622, -0.9466) centre (-29.7621, -2) ccw projected
  line L3 (-31.4622, -0.9466) -> (-38.4435, -12.2139) projected
  arc A2 (-38.4435, -12.2139) -> (-39.943, -17.4809) centre (-29.943, -17.4809) ccw projected
  line L4 (-39.943, -17.4809) -> (-39.943, -23.7301) projected
  line L5 (-39.943, -23.7301) -> (32.5965, -23.7301) projected
  line L6 (32.5965, -23.7301) -> (40.9756, -20.8275) projected
  circle A3 centre (4.5999, -15.7301) radius 4.1 projected
  circle A4 centre (25.5999, -5.7301) radius 4.1 projected
  point P0 (12.8122, 9.1135)
extrude "Extrusion58" add sketch "Sketch59" against normal up to surface (13.6342 mm away) contours A3
sketch "Sketch60" plane through (41.5818, -9.1135, -5.4793) normal (0, 0, 1) x (1, 0, 0)
  circle A0 centre (-33.3695, -15.7301) radius 4.1 projected
  point P0 (-41.5818, 9.1135)
extrude "Extrusion59" add sketch "Sketch60" against normal up to surface (13.6342 mm away)
sketch "Sketch61" plane through (0, 0, 0) normal (-1, 0, 0) x (0, 0, 1)
  line L0 (-84.7477, -9.1135) -> (-39.9593, -9.1135) projected
  arc A0 (-40.9593, -8.1135) -> (-39.9593, -9.1135) centre (-39.9593, -8.1135) ccw projected
  line L1 (-40.9593, -8.1135) -> (-40.9593, 16.2865) projected
  line L2 (-40.9593, 16.2865) -> (-53.9593, 16.2865) projected
  line L3 (-53.9593, 16.2865) -> (-84.7477, -9.1135) projected
  point P0 (0, 0)
extrude "Extrusion60" add sketch "Sketch61" along normal up to surface round surface about axis through (-97.9498, 22.4842, -84.7477) along (0, 0, 1) radius 87.2843 far side no
sketch "Sketch62" plane through (52.7552, -32.8436, -84.7477) normal (0, 0, -1) x (-1, 0, 0)
  arc A0 (63.641, 49.1301) -> (69.3408, 23.7301) centre (150.705, 55.3278) ccw projected
  arc A1 (69.3408, 23.7301) -> (80.9186, 2.9026) centre (150.705, 55.3278) ccw projected
  arc A2 (73.5118, 14.5877) -> (92.7552, -9.9437) centre (150.705, 55.3278) ccw projected
  arc A3 (63.641, 49.1301) -> (92.7552, -9.9437) centre (150.705, 55.3278) ccw
  line L0 (57.0451, 49.1301) -> (90.2775, -20.9598)
  line L1 (39.943, 23.7301) -> (39.943, 49.1301) projected
  line L2 (39.943, 23.7301) -> (69.3408, 23.7301) projected
  arc A4 (63.641, 49.1301) -> (69.3408, 23.7301) centre (150.705, 55.3278) ccw projected
  line L3 (39.943, 49.1301) -> (63.641, 49.1301) projected
  arc A5 (73.5118, 14.5877) -> (92.7552, -9.9437) centre (150.705, 55.3278) ccw projected
  line L4 (73.5118, 14.5877) -> (21.8108, 14.5877) projected
  arc A6 (21.8108, 14.5877) -> (16.5429, 13.0877) centre (21.8108, 4.5877) ccw projected
  arc A7 (16.5429, 13.0877) -> (3.4552, 0) centre (16.5429, 0) ccw projected
  line L5 (3.4552, 0) -> (0, 0) projected
  line L6 (0, -5.2586) -> (0, 0) projected
  arc A8 (0, -5.2586) -> (7.4723, -14.9338) centre (10, -5.2586) ccw projected
  line L7 (7.4723, -14.9338) -> (67.6998, -30.6683) projected
  arc A9 (67.6998, -30.6683) -> (92.7552, -11.3177) centre (72.7552, -11.3177) ccw projected
  line L8 (92.7552, -9.9437) -> (92.7552, -11.3177) projected
  circle A10 centre (16.5429, 0) radius 11 projected
  circle A11 centre (68.4659, -14.233) radius 11.1 projected
  point P0 (52.7552, 32.8436)
  point P1 (92.7552, -9.9437)
  point P2 (73.5118, 14.5877)
  point P3 (73.423, 14.5877)
  point P4 (63.641, 49.1301)
  point P5 (69.0883, 23.7301)
  point P6 (69.3408, 23.7301)
  point P7 (71.8367, 17.9333)
  point P8 (69.3408, 23.7301)
  constraints: 4 end point, 4 point on circle, 1 centre point, 1 coincident, 1 point on line, 1 tangent
extrude "Extrusion61" cut sketch "Sketch62" against normal through all contours A1 L4 L0 | A0 L2 L0 L3 | A1 L0 L2 | A1 A2 L8 A9 L0 L4
body "Solid1"
